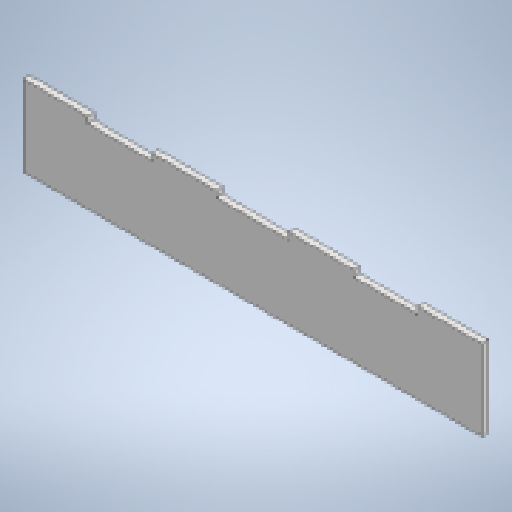
# Autodesk Inventor part: стенкаB
Saved by Autodesk Inventor 2023 (Build 270158000, 158)
## iProperties
Created: 2025-02-04
Part Number: стенкаB
Material: Типовые
Document SubType Name: Modeling
Designer: baranovaem
Density: 1 g/cm^3
Appearance: По умолчанию
Author: baranovaem
Autodesk Inventor part; units mm, degrees
ref_plane "YZ Plane" through (0, 0, 0) normal (1, 0, 0) x (0, 1, 0)
ref_plane "XZ Plane" through (0, 0, 0) normal (0, 1, 0) x (-1, 0, 0)
ref_plane "XY Plane" through (0, 0, 0) normal (0, 0, 1) x (1, 0, 0)
sketch "Эскиз1" plane through (0, 0, 0) normal (0, 0, 1) x (1, 0, 0)
  line L0 (-142.5, 23) -> (142.5, 23)
  line L1 (142.5, 23) -> (142.5, -23)
  line L2 (142.5, -23) -> (-142.5, -23)
  line L3 (-142.5, -23) -> (-142.5, 23)
  line L4 (-142.5, 23) -> (142.5, -23) construction
  line L5 (142.5, 23) -> (-142.5, -23) construction
  point P0 (0, 0)
  dimension "d0" = 285
  dimension "d1" = 46
  constraints: 12 end point, 2 midpoint, 2 parallel, 1 horizontal, 1 perpendicular
  measures "d0" distance of L1.end L2.end
  measures "d1" distance of L0.end L1.end
extrude "Выдавливание1" add sketch "Эскиз1" along normal blind 4
sketch "Эскиз2" plane through (-142.5, 23, 0) normal (0, 1, 0) x (1, 0, 0)
  line L0 (285, 0) -> (0, 0) projected
  line L1 (0, 0) -> (0, -4) projected
  line L2 (285, -4) -> (0, -4) projected
  line L3 (285, 0) -> (285, -4) projected
  line L4 (40, 0) -> (40, -4)
  line L5 (0, 0) -> (285, 0) projected
  line L6 (80, 0) -> (80, -4)
  line L7 (165, 0) -> (165, -4)
  line L8 (0, -4) -> (285, -4) projected
  line L9 (205, 0) -> (205, -4)
  line L10 (245, 0) -> (245, -4)
  line L11 (120, -4) -> (120, 0)
  point P0 (142.5, 0)
  point P1 (0, -2)
  point P2 (40, -2)
  point P3 (285, -2)
  point P4 (165, -2)
  point P5 (205, -2)
  point P6 (245, -2)
  point P7 (80, -2)
  point P8 (120, -2)
  dimension "d4" = 40
  dimension "d5" = 40
  dimension "d6" = 40
  dimension "d8" = 40
  dimension "d9" = 40
  dimension "d10" = 40
  constraints: 12 end point, 12 point on line, 8 midpoint, 4 perpendicular, 1 parallel, 1 vertical
  measures "d4" distance of point (0, -2) point (40, -2)
  measures "d5" horizontal distance of point (285, -2) L10.start
  measures "d6" distance of point (165, -2) point (205, -2)
  measures "d8" distance of point (80, -2) point (120, -2)
  measures "d9" distance of point (80, -2) point (40, -2)
  measures "d10" distance of point (245, -2) point (205, -2)
extrude "Выдавливание2" add sketch "Эскиз2" along normal blind 4 contours L3 L2 L10 L0 | L9 L2 L7 L0 | L11 L2 L6 L0 | L4 L2 L1 L0
